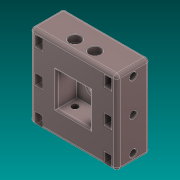
# Autodesk Inventor part: plaathouder en koppeling axis 4_5
Saved by Autodesk Inventor 2020 (Build 240168000, 168)
## iProperties
Created: 2020-05-27
Part Number: plaathouder en koppeling axis 4_5
Material: ABS Plastic
Document SubType Name: Modeling
Designer: stefa
Density: 1.06 g/cm^3
Appearance: Smooth - White
Author: stefa
Autodesk Inventor part; units mm, degrees
ref_plane "YZ Plane" through (0, 0, 0) normal (1, 0, 0) x (0, 1, 0)
ref_plane "XZ Plane" through (0, 0, 0) normal (0, 1, 0) x (-1, 0, 0)
sketch "Sketch1" plane through (0, 0, 0) normal (0, 0, 1) x (1, 0, 0)
  line L0 (-26, -25) -> (26, -25)
  line L1 (26, -25) -> (26, 25)
  line L2 (26, 25) -> (-26, 25)
  line L3 (-26, 25) -> (-26, -25)
  line L4 (-26, -25) -> (26, 25) construction
  line L5 (26, -25) -> (-26, 25) construction
  point P0 (0, 0)
  dimension "d0" = 52
  dimension "d1" = 50
  constraints: 12 end point, 2 midpoint, 2 parallel, 1 horizontal, 1 perpendicular
  measures "d0" distance of L2.end L1.end
  measures "d1" distance of L1.end L0.end
extrude "Extrusion1" add sketch "Sketch1" along normal mid plane 20
sketch "Sketch2" plane through (26, -25, -10) normal (1, 0, 0) x (0, 0, -1)
  circle A0 centre (-10, 5) radius 2.05
  line L0 (0, 50) -> (0, 0) projected
  line L1 (0, 0) -> (-20, 0) projected
  circle A1 centre (-10, 25) radius 2.05
  circle A2 centre (-10, 45) radius 2.05
  dimension "d4" = 4.1
  dimension "d5" = 10
  dimension "d6" = 5
  dimension "d7" = 50
  dimension "d8" = 20
  dimension "d21" = 0
  dimension "d51" = 20
  constraints: 3 centre point, 2 equal radius, 2 vertical alignment, 1 other
  measures "d4" diameter of A0
  measures "d6" distance from line of L1 A0.centre
  measures "d7" distance of L1.start point (0, 50)
  measures "d8" distance of L1.start L1.end
  measures "d21" distance of A0.centre point (-10, 5)
  measures "d51" distance of A0.centre A1.centre
sketch "Sketch3" plane through (0, 0, 10) normal (0, 0, 1) x (1, 0, 0)
  circle A0 centre (0, 0) radius 4
  line L0 (-10, -10) -> (10, -10)
  line L1 (10, -10) -> (10, 10)
  line L2 (10, 10) -> (-10, 10)
  line L3 (-10, 10) -> (-10, -10)
  line L4 (-10, -10) -> (10, 10) construction
  line L5 (10, -10) -> (-10, 10) construction
  dimension "d31" = 8
  dimension "d32" = 20
  dimension "d33" = 20
  constraints: 12 end point, 2 midpoint, 2 parallel, 1 centre point, 1 coincident, 1 horizontal, 1 perpendicular
  measures "d31" diameter of A0
  measures "d32" distance of L1.end L2.end
  measures "d33" distance of L0.end L1.end
extrude "Extrusion2" cut sketch "Sketch3" against normal through all contours A0
extrude "Extrusion3" cut sketch "Sketch3" against normal blind 12
sketch "Sketch4" plane through (-26, -25, -10) normal (0, -1, 0) x (1, 0, 0)
  circle A0 centre (20, 13) radius 2.05
  line L0 (52, 0) -> (0, 0) projected
  line L1 (26, 10) -> (26, 20) construction
  circle A1 centre (20, 13) radius 3.5
  circle A2 centre (32, 13) radius 2.05
  circle A3 centre (32, 13) radius 3.5
  line L2 (0, 20) -> (52, 20) projected
  dimension "d38" = 4.1
  dimension "d40" = 6
  dimension "d42" = 7
  dimension "d48" = 7
  constraints: 4 centre point, 2 coincident, 2 end point, 2 symmetric about line, 1 midpoint, 1 vertical, 3 other
  measures "d38" diameter of A0
  measures "d40" horizontal distance of L1.start A0.centre
  measures "d42" diameter of A1
  measures "d48" distance from line of L2 A0.centre
extrude "Extrusion4" cut sketch "Sketch4" against normal blind 4.1
extrude "Extrusion5" cut sketch "Sketch4" against normal up to surface (15 mm away) contours A0 | A2
mirror "Mirror1" about plane through (0, 0, 0) normal (0, 1, 0) of "Extrusion4", "Extrusion5"
extrude "Extrusion6" cut sketch "Sketch2" against normal blind 12
ref_plane "Work Plane1" through (23, -25, 10) normal (1, 0, 0) x (0, 0, -1)
sketch "Sketch6" plane through (23, -25, 10) normal (1, 0, 0) x (0, 0, -1)
  line L0 (10.5, 4.1) -> (3.5, 4.1) projected
  line L1 (6.1779, 4.1) -> (8.089, 7.41)
  line L2 (8.089, 7.41) -> (11.911, 7.41)
  line L3 (11.911, 7.41) -> (13.8221, 4.1)
  line L4 (13.8221, 4.1) -> (11.911, 0.79)
  line L5 (11.911, 0.79) -> (8.089, 0.79)
  line L6 (8.089, 0.79) -> (6.1779, 4.1)
  line L7 (8.089, 0.79) -> (0, 0.79)
  line L8 (0, 50) -> (0, 0) projected
  line L9 (8.089, 7.41) -> (0, 7.41)
  line L10 (8.089, 27.41) -> (0, 27.41)
  line L11 (8.089, 20.79) -> (0, 20.79)
  line L12 (8.089, 20.79) -> (6.1779, 24.1)
  line L13 (11.911, 20.79) -> (8.089, 20.79)
  line L14 (13.8221, 24.1) -> (11.911, 20.79)
  line L15 (11.911, 27.41) -> (13.8221, 24.1)
  line L16 (8.089, 27.41) -> (11.911, 27.41)
  line L17 (6.1779, 24.1) -> (8.089, 27.41)
  line L18 (8.089, 47.41) -> (0, 47.41)
  line L19 (8.089, 40.79) -> (0, 40.79)
  line L20 (8.089, 40.79) -> (6.1779, 44.1)
  line L21 (11.911, 40.79) -> (8.089, 40.79)
  line L22 (13.8221, 44.1) -> (11.911, 40.79)
  line L23 (11.911, 47.41) -> (13.8221, 44.1)
  line L24 (8.089, 47.41) -> (11.911, 47.41)
  line L25 (6.1779, 44.1) -> (8.089, 47.41)
  point P0 (10, 25)
  point P1 (10, 4.1)
  point P2 (10, 24.1)
  point P3 (10, 44.1)
  dimension "d59" = 6.62
  dimension "d62" = 20
  dimension "d67" = 20
  constraints: 48 end point, 4 point on line, 1 horizontal, 1 parallel, 1 vertical, 1 vertical alignment, 47 other
  measures "d59" distance between parallel lines of L2 L5
  measures "d62" distance of L1.end L10.start
  measures "d67" distance of point (10, 24.1) point (10, 4.1)
extrude "Extrusion7" cut sketch "Sketch6" against normal blind 4.6
mirror "Mirror3" about plane through (0, 0, 0) normal (1, 0, 0) of "Extrusion7", "Extrusion6"
fillet "Fillet1" radius 2 4 edges at (26, -25, 0) (-26, -25, 0) (26, 25, 0) (-26, 25, 0)
fillet "Fillet2" radius 2 16 edges at (25.4142, -24.4142, 10) (26, 0, 10) (25.4142, 24.4142, 10) (0, 25, 10) (-25.4142, 24.4142, 10) (-26, 0, 10) (-25.4142, -24.4142, 10) (0, -25, 10) (-25.4142, -24.4142, -10) (-26, 0, -10) (-25.4142, 24.4142, -10) (0, 25, -10) (25.4142, 24.4142, -10) (26, 0, -10) (25.4142, -24.4142, -10) (0, -25, -10)
fillet "Fillet3" radius 1 4 edges at (-10, 0, 10) (0, 10, 10) (10, 0, 10) (0, -10, 10)
fillet "Fillet4" radius 0.2 12 edges at (10.2929, 10.2929, 9.7071) (10, 10, 3.5) (-10.2929, 10.2929, 9.7071) (-10, 10, 3.5) (10.2929, -10.2929, 9.7071) (10, -10, 3.5) (-10.2929, -10.2929, 9.7071) (-10, -10, 3.5) (-10, 0, -2) (0, 10, -2) (10, 0, -2) (0, -10, -2)
fillet "Fillet5" radius 1 2 edges at (-4, 0, -2) (-4, 0, -10)
chamfer "Chamfer1" distance 0.3 angle 45 10 edges at (26, -20, 2.05) (26, 0, 2.05) (26, 20, 2.05) (2.5, 25, 3) (-9.5, 25, 3) (-26, 20, 2.05) (-26, 0, 2.05) (-26, -20, 2.05) (-9.5, -25, 3) (2.5, -25, 3)
equation "\"d21\" = d8 - 2 * d5"
body "Solid1"
